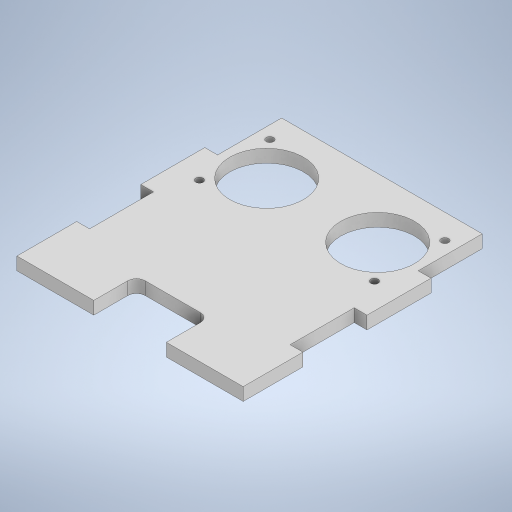
# Autodesk Inventor part: do_sensor_1_3mm
Saved by Autodesk Inventor 2023 (Build 270158000, 158)
## iProperties
Created: 2022-11-21
Part Number: do_sensor_1_3mm
Material: Generic
Document SubType Name: Modeling
Designer: ADMIN
Density: 1 g/cm^3
Appearance: Default
Author: ADMIN
Autodesk Inventor part; units mm, degrees
ref_plane "YZ Plane" through (0, 0, 0) normal (1, 0, 0) x (0, 1, 0)
ref_plane "XZ Plane" through (0, 0, 0) normal (0, 1, 0) x (-1, 0, 0)
ref_plane "XY Plane" through (0, 0, 0) normal (0, 0, 1) x (1, 0, 0)
sketch "Sketch1" plane through (0, 0, 0) normal (0, 1, 0) x (-1, 0, 0)
  circle A0 centre (-7.5, 8.25) radius 0.875
  circle A1 centre (-7.5, -8.25) radius 0.875
  circle A2 centre (33.5, 8.25) radius 0.875
  circle A3 centre (33.5, -8.25) radius 0.875
  circle A4 centre (0, 0) radius 8.6279
  circle A5 centre (26, 0) radius 8.6279
  line L0 (-13.5, -14) -> (36.5, -14)
  line L1 (39.5, 45) -> (21.5, 45)
  line L2 (21.5, 45) -> (21.5, 37)
  line L3 (4.5, 45) -> (4.5, 37)
  line L4 (19.5, 35) -> (6.5, 35)
  line L5 (39.5, 45) -> (21.5, 45)
  line L6 (4.5, 45) -> (-13.5, 45)
  line L7 (-13.5, 45) -> (39.285, 45) construction
  arc A6 (19.5, 35) -> (21.5, 37) centre (19.5, 37) ccw
  arc A7 (4.5, 37) -> (6.5, 35) centre (6.5, 37) ccw
  line L8 (-10.5, -14) -> (-10.5, 1)
  line L9 (-10.5, 1) -> (-13.5, 1)
  line L10 (-13.5, 1) -> (-13.5, 16)
  line L11 (-13.5, 16) -> (-10.5, 16)
  line L12 (-10.5, 16) -> (-10.5, 31)
  line L13 (-10.5, 31) -> (-13.5, 31)
  line L14 (-13.5, 45) -> (-13.5, 31)
  line L15 (-13.5, 16) -> (-13.5, 1)
  line L16 (36.5, -14) -> (36.5, 1)
  line L17 (36.5, 1) -> (39.5, 1)
  line L18 (39.5, 16) -> (36.5, 16)
  line L19 (36.5, 16) -> (36.5, 31)
  line L20 (36.5, 31) -> (39.5, 31)
  line L21 (39.5, 1) -> (39.5, 16)
  line L22 (39.5, 31) -> (39.5, 45)
  point P0 (35.5, -10)
  point P1 (21.5, 35)
  dimension "d5" = 1.75
  dimension "d6" = 1.75
  dimension "d7" = 1.75
  dimension "d8" = 1.75
  dimension "d11" = 18
  dimension "d12" = 10
  dimension "d14" = 2
  dimension "d15" = 3
  dimension "d17" = 15
  dimension "d18" = 15
  constraints: 46 end point, 9 perpendicular, 8 centre point, 6 parallel, 4 point on circle, 4 tangent, 3 point on line, 1 equal radius, 1 horizontal, 1 vertical
  measures "d5" diameter of A0
  measures "d6" diameter of A1
  measures "d7" diameter of A2
  measures "d8" diameter of A3
  measures "d11" distance of L1.start L1.end
  measures "d12" distance of L1.end point (21.5, 35)
  measures "d14" radius of A6
  measures "d15" distance of L0.start L8.start
  measures "d17" distance of L9.end L10.end
  measures "d18" distance of L11.end L12.end
extrude "Extrusion1" add sketch "Sketch1" along normal blind 3
body "Solid1"
